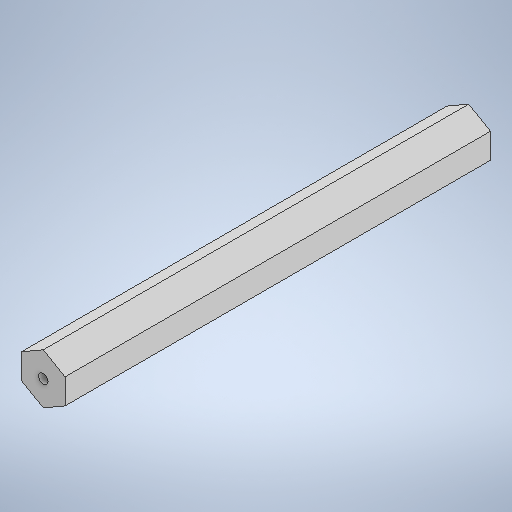
# Autodesk Inventor part: TheHandleBar
Saved by Autodesk Inventor 2025.1 (Build 291241000, 241)
## iProperties
Created: 2026-05-11
Part Number: TheHandleBar
Material: Generic
Document SubType Name: Modeling
Designer: User
Density: 1 g/cm^3
Appearance: Default
Author: User
## iProperties of the stored document TheHandleBar_3DPrint.ipt
Created: 2026-05-12
Part Number: TheHandleBar_3DPrint
Material: Generic
Document SubType Name: Modeling
Designer: User
Density: 1 g/cm^3
Appearance: Default
Author: User
Autodesk Inventor part; units mm, degrees
ref_plane "YZ Plane" through (0, 0, 0) normal (1, 0, 0) x (0, 1, 0)
ref_plane "XZ Plane" through (0, 0, 0) normal (0, 1, 0) x (-1, 0, 0)
sketch "Sketch1" plane through (0, 0, 0) normal (0, 0, 1) x (1, 0, 0)
  circle A0 centre (-0.0005, 100.4366) radius 2.5 projected
  arc A1 (7.4995, 100.4366) -> (-7.5005, 100.4366) centre (-0.0005, 100.4366) ccw projected
  circle A2 centre (-0.0005, 100.4366) radius 7.5
  arc A3 (11.4995, 100.4366) -> (-11.5005, 100.4365) centre (-0.0005, 100.4366) ccw projected
  circle A4 centre (-0.0005, 100.4366) radius 11.5
  line L0 (-0.0005, 100.4366) -> (11.4995, 107.0761)
  line L1 (-0.0005, 100.4366) -> (16.6776, 100.4366) construction
  line L2 (-0.0005, 111.9366) -> (9.9588, 106.1866)
  line L3 (5.7495, 110.3959) -> (4.9792, 109.0616)
  line L4 (-0.0005, 113.7156) -> (11.4995, 107.0761)
  line L5 (-4.6563, 116.4037) -> (19.5852, 116.4037) construction
  line L6 (-0.0005, 100.4366) -> (-0.0005, 113.7156)
  line L7 (-11.5005, 107.0761) -> (-0.0005, 113.7156)
  line L8 (-11.5005, 93.7971) -> (-11.5005, 107.0761)
  line L9 (-0.0005, 87.1575) -> (-11.5005, 93.7971)
  line L10 (11.4995, 93.7971) -> (-0.0005, 87.1575)
  line L11 (11.4995, 107.0761) -> (11.4995, 93.7971)
  point P0 (0, 0)
  point P1 (11.4995, 100.4366)
  point P2 (11.4995, 100.4366)
  dimension "d0" = 30
  dimension "d1" = 30
  dimension "d4" = 360
  constraints: 24 end point, 3 point on circle, 2 centre point, 2 coincident, 2 concentric, 2 horizontal, 2 point on line, 1 midpoint, 1 perpendicular, 1 tangent, 1 vertical, 19 other
  measures "d0" angle of L1 L0
  measures "d1" angle of L4 L5
ref_plane "Work Plane1" through (-7.5007, -7.5, 224.8016) normal (0, 0, -1) x (0, 1, 0)
extrude "Extrusion1" add sketch "Sketch1" along normal up to surface (224.8016 mm away) contours A0 L0 A1 A2 L6 | A0 L6 A1 L0 | L0 A3 A4 L6 A1 A2 | A1 L6 L2 L0 | L0 L11 A3 | L2 L3 A3 | A3 L4 L0 | L6 L4 A3 | A3 L3 L2 | A3 L7 L6 | L11 L10 A4 | A3 L8 L7 | L10 L9 A4 | A4 L9 L8
body "Solid1"
